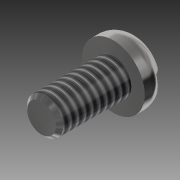
# Autodesk Inventor part: M3x10 Screw Nylon
Saved by Autodesk Inventor 2015 (Build 190159000, 159)
## iProperties
Created: 2016-02-18
Part Number: M3x10 Screw Nylon
Material: Steel
Document SubType Name: Modeling
Designer: 23902
Density: 7.85 g/cm^3
Appearance: Plate
Mass: 0.113453 g
Surface Area: 1.50413 cm^2
Volume: 0.101298 cm^3
Author: 23902
Autodesk Inventor part; units mm, degrees
ref_plane "YZ Plane" through (0, 0, 0) normal (1, 0, 0) x (0, 1, 0)
ref_plane "XZ Plane" through (0, 0, 0) normal (0, 1, 0) x (-1, 0, 0)
ref_plane "XY Plane" through (0, 0, 0) normal (0, 0, 1) x (1, 0, 0)
sketch "Sketch1" plane through (0, 0, 0) normal (0, 1, 0) x (-1, 0, 0)
  circle A0 centre (0, 0) radius 1
  dimension "d0" = 2
  constraints: 1 centre point, 1 coincident
  measures "d0" diameter of A0
extrude "Extrusion1" add sketch "Sketch1" along normal blind 4
sketch "Sketch2" plane through (0, 4, 0) normal (0, 1, 0) x (1, 0, 0)
  circle A0 centre (0, 0) radius 1.75
  dimension "d3" = 3.5
  constraints: 1 centre point, 1 coincident
  measures "d3" diameter of A0
extrude "Extrusion2" add sketch "Sketch2" along normal blind 1.4
thread "Thread2" size "M2x0.4" class "6g" standard "ANSI Metric M Profile" full length
chamfer "Chamfer2" distance 0.2 angle 45 1 edges at (1, 0, 0)
fillet "Fillet2" radius 1 1 edges at (-1.75, 5.4, 0)
sketch "Sketch4" plane through (0, 5.4, 0) normal (0, 1, 0) x (1, 0, 0)
  line L0 (-1.758, -0.5) -> (1.758, -0.5)
  line L1 (1.758, -0.5) -> (1.758, 0.5)
  line L2 (1.758, 0.5) -> (-1.758, 0.5)
  line L3 (-1.758, 0.5) -> (-1.758, -0.5)
  line L4 (-1.758, -0.5) -> (1.758, 0.5) construction
  line L5 (1.758, -0.5) -> (-1.758, 0.5) construction
  line L6 (-0.5, -1.25) -> (-0.5, 1.25)
  line L7 (-0.5, 1.25) -> (0.5, 1.25)
  line L8 (0.5, 1.25) -> (0.5, -1.25)
  line L9 (0.5, -1.25) -> (-0.5, -1.25)
  circle A0 centre (0, 0) radius 1.75 projected
  line L10 (-0.5, -1.25) -> (0.5, 1.25) construction
  line L11 (-0.5, 1.25) -> (0.5, -1.25) construction
  dimension "d23" = 1
  dimension "d24" = 2.5
  dimension "d25" = 1
  constraints: 24 end point, 5 parallel, 4 midpoint, 2 perpendicular, 1 horizontal
  measures "d23" distance of L1.end L0.end
  measures "d24" distance of L6.start L6.end
  measures "d25" distance of L6.end L7.end
extrude "Extrusion4" cut sketch "Sketch4" against normal blind 0.6 contours L3 L2 A0 L0 | A0 L2 L6 L0 | L6 L2 L8 L0 | L0 L8 L9 L6 | A0 L2 L1 L0 | L0 L8 L2 A0 | L6 L7 L8 L2
body "Solid1"
